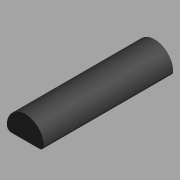
# Autodesk Inventor part: Part1
Saved by Autodesk Inventor 2019.3 (Build 233278000, 278)
## iProperties
Part Number: Part1
Material: Generic
Document SubType Name: Modeling
Designer: Frienddo
Appearance: Default
Author: Frienddo
Autodesk Inventor part; units mm, degrees
ref_plane "YZ Plane" through (0, 0, 0) normal (1, 0, 0) x (0, 1, 0)
ref_plane "XZ Plane" through (0, 0, 0) normal (0, 1, 0) x (-1, 0, 0)
ref_plane "XY Plane" through (0, 0, 0) normal (0, 0, 1) x (1, 0, 0)
sketch "Sketch1" plane through (0, 0, 0) normal (0, 0, 1) x (1, 0, 0)
  arc A0 (20, 0) -> (-20, 0) centre (0, 0) ccw
  line L0 (-20, 0) -> (-20, 0)
  line L1 (-15, -5) -> (15, -5)
  line L2 (20, 0) -> (20, 0)
  arc A1 (-20, 0) -> (-15, -5) centre (-15, 0) ccw
  arc A2 (15, -5) -> (20, 0) centre (15, 0) ccw
  point P0 (-20, -5)
  point P1 (20, -5)
  dimension "d0" = 40
  dimension "d1" = 20
  dimension "d2" = 5
  dimension "d5" = 5
  dimension "d6" = 5
  constraints: 6 end point, 6 point on circle, 4 point on line, 4 tangent, 3 centre point, 2 perpendicular, 1 coincident, 1 vertical
  measures "d0" distance of point (-20, -5) point (20, -5)
  measures "d1" radius of A0
  measures "d2" distance from line of L2.end L1
  measures "d5" radius of A1
  measures "d6" radius of A2
extrude "Extrusion1" add sketch "Sketch1" along normal mid plane 140
body "Solid1"
